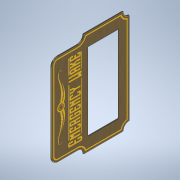
# Autodesk Inventor part: EW_MessingplatteUhrzeit
Saved by Autodesk Inventor 2020 (Build 240168000, 168)
## iProperties
Created: 2020-06-21
Part Number: EW_MessingplatteUhrzeit
Material: Messing
Document SubType Name: Modeling
Designer: Johannes
Density: 8.49 g/cm^3
Appearance: Messing - satiniert 1
Author: Johannes
Autodesk Inventor part; units mm, degrees
ref_plane "YZ Plane" through (0, 0, 0) normal (1, 0, 0) x (0, 1, 0)
ref_plane "XZ Plane" through (0, 0, 0) normal (0, 1, 0) x (-1, 0, 0)
ref_plane "XY Plane" through (0, 0, 0) normal (0, 0, 1) x (1, 0, 0)
sketch "Skizze1" plane through (0, 0, 0) normal (1, 0, 0) x (0, 1, 0)
  line L0 (-50, -37.5) -> (50, -37.5)
  line L1 (50, -37.5) -> (50, 37.5)
  line L2 (50, 37.5) -> (-50, 37.5)
  line L3 (-50, 37.5) -> (-50, -37.5)
  line L4 (-50, -37.5) -> (50, 37.5) construction
  line L5 (50, -37.5) -> (-50, 37.5) construction
  point P0 (0, 0)
  dimension "d0" = 100
  dimension "d1" = 75
  constraints: 12 end point, 2 midpoint, 2 parallel, 1 horizontal, 1 perpendicular
  measures "d0" distance of L2.end L1.end
  measures "d1" distance of L1.end L0.end
extrude "Extrusion1" add sketch "Skizze1" along normal blind 0.8
sketch "Skizze2" plane through (0.8, 0, 0) normal (1, 0, 0) x (0, 0, -1)
  line L0 (-37.5, -50) -> (-6.5, -50)
  line L1 (-6.5, -50) -> (-6.5, -44)
  line L2 (-6.5, -44) -> (-37.5, -44)
  line L3 (-37.5, -44) -> (-37.5, -50)
  line L4 (-37.5, 50) -> (-6.5, 50)
  line L5 (-6.5, 50) -> (-6.5, 44)
  line L6 (-6.5, 44) -> (-37.5, 44)
  line L7 (-37.5, 44) -> (-37.5, 50)
  line L8 (31.5, -50) -> (37.5, -50)
  line L9 (37.5, -50) -> (37.5, -44)
  line L10 (37.5, -44) -> (31.5, -44)
  line L11 (31.5, -44) -> (31.5, -50)
  line L12 (37.5, 50) -> (31.5, 50)
  line L13 (31.5, 50) -> (31.5, 44)
  line L14 (31.5, 44) -> (37.5, 44)
  line L15 (37.5, 44) -> (37.5, 50)
  line L16 (-2.5, -37.5) -> (27.5, -37.5)
  line L17 (27.5, -37.5) -> (27.5, 37.5)
  line L18 (27.5, 37.5) -> (-2.5, 37.5)
  line L19 (-2.5, 37.5) -> (-2.5, -37.5)
  line L20 (52.5, 0) -> (-52.5, 0) construction
  line L21 (-37.5, 50) -> (-37.5, -50) construction
  point P0 (0, 0)
  dimension "d4" = 6
  dimension "d5" = 6
  dimension "d6" = 31
  dimension "d9" = 75
  dimension "d10" = 30
  dimension "d11" = 35
  constraints: 40 end point, 10 parallel, 5 collinear, 5 horizontal, 5 perpendicular, 4 coincident, 1 other
  measures "d4" distance of L0.end L1.end
  measures "d5" distance of L9.end L10.end
  measures "d6" distance of L1.end L2.end
  measures "d9" distance of L18.end L16.start
  measures "d10" distance of L16.start L16.end
  measures "d11" distance between parallel lines of L21 L19
extrude "Extrusion2" cut sketch "Skizze2" against normal through all
fillet "Rundung1" radius 6 6 edges at (0.4, -44, 6.5) (0.4, -44, -31.5) (0.4, 44, -31.5) (0.4, 44, 6.5) (0.4, 44, 37.5) (0.4, -44, 37.5)
fillet "Rundung1" radius 0.5 4 edges at (0.4, -37.5, 2.5) (0.4, -37.5, -27.5) (0.4, 37.5, -27.5) (0.4, 37.5, 2.5)
sketch "Skizze3" plane through (0.8, 0, 0) normal (1, 0, 0) x (0, 0, -1)
  line L0 (-37.5, 50) -> (95.7584, 50) construction
  line L1 (95.7584, 50) -> (95.7584, -50) construction
  line L2 (95.7584, -50) -> (-37.5, -50) construction
  line L3 (-37.5, -50) -> (-37.5, 50) construction
  line L4 (-6.5, -50) -> (31.5, -50) projected
  line L5 (-37.5, 38) -> (-37.5, -38) projected
  point P0 (0, 0)
  dimension "d26" = 100
  constraints: 2 collinear, 2 other
  measures "d26" distance of L2.end L0.start
decal "Aufkleber1"
